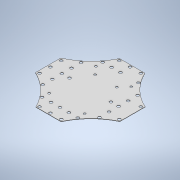
# Autodesk Inventor part: pixfalcon_acc_board_light
Saved by Autodesk Inventor 2020 (Build 240168000, 168)
## iProperties
Created: 2019-06-13
Part Number: pixfalcon_acc_board_light
Material: Generic
Document SubType Name: Modeling
Designer: amirt
Density: 1 g/cm^3
Appearance: Default
Author: amirt
Autodesk Inventor part; units mm, degrees
ref_plane "YZ Plane" through (0, 0, 0) normal (1, 0, 0) x (0, 1, 0)
ref_plane "XZ Plane" through (0, 0, 0) normal (0, 1, 0) x (-1, 0, 0)
ref_plane "XY Plane" through (0, 0, 0) normal (0, 0, 1) x (1, 0, 0)
sketch "Sketch1" plane through (25.3999, 76.2, 1203.3249) normal (0, 1, 0) x (-1, 0, 0)
  circle A0 centre (-1238.2523, -1095.3736) radius 57.1474 projected
  circle A1 centre (-1670.051, -1095.3758) radius 57.1513 projected
  circle A2 centre (-958.8491, -714.3774) radius 57.1526 projected
  circle A3 centre (-1314.4507, -714.3762) radius 57.1514 projected
  circle A4 centre (-1670.0504, -714.3731) radius 57.1481 projected
  circle A5 centre (-2101.8571, -1095.3735) radius 57.1571 projected
  circle A6 centre (-2381.2539, -714.3704) radius 57.1441 projected
  circle A7 centre (-2374.9001, -437.5189) radius 44.4462 projected
  circle A8 centre (-965.201, -437.5113) radius 44.4463 projected
  circle A9 centre (-1238.2504, -135.2557) radius 44.4509 projected
  circle A10 centre (-539.7501, -269.8758) radius 57.1508 projected
  circle A11 centre (-82.5498, 60.325) radius 57.1503 projected
  circle A12 centre (-82.5503, 492.1251) radius 57.1497 projected
  circle A13 centre (-82.5503, 923.9249) radius 57.1497 projected
  circle A14 centre (-539.7506, 1254.1242) radius 57.149 projected
  circle A15 centre (-539.7506, 873.1259) radius 57.149 projected
  circle A16 centre (-539.7488, 492.1268) radius 57.1522 projected
  circle A17 centre (-539.7501, 111.124) radius 57.151 projected
  circle A18 centre (-844.552, 492.1153) radius 57.1402 projected
  circle A19 centre (-965.2029, 1421.7493) radius 44.4342 projected
  circle A20 centre (-958.8546, 1698.6268) radius 57.1451 projected
  circle A21 centre (-1238.2501, 2079.6258) radius 57.1505 projected
  circle A22 centre (-1314.4494, 1698.6235) radius 57.1516 projected
  circle A23 centre (-1670.0494, 1698.6235) radius 57.1516 projected
  circle A24 centre (-2025.6555, 1698.6281) radius 57.1438 projected
  circle A25 centre (-2381.2575, 1698.6334) radius 57.1389 projected
  circle A26 centre (-2101.8503, 2079.6254) radius 57.1496 projected
  circle A27 centre (-1670.0543, 2079.6363) radius 57.1384 projected
  circle A28 centre (-2374.8997, 1421.7644) radius 44.4506 projected
  circle A29 centre (-2800.3552, 1254.1333) radius 57.1404 projected
  circle A30 centre (-3257.5497, 923.9267) radius 57.1482 projected
  circle A31 centre (-2800.3372, 873.132) radius 57.1356 projected
  circle A32 centre (-2495.5435, 492.1228) radius 57.157 projected
  circle A33 centre (-2800.3503, 492.134) radius 57.1411 projected
  circle A34 centre (-3257.5494, 60.3259) radius 57.1489 projected
  circle A35 centre (-2800.342, 111.1204) radius 57.1592 projected
  circle A36 centre (-2800.3554, -269.8798) radius 57.1572 projected
  circle A37 centre (-2101.8507, -135.2543) radius 44.4491 projected
  line L0 (-82.5503, 930.2676) -> (-82.5503, 923.9249)
  line L1 (22.2091, 981.2172) -> (-3340.1002, 981.2172)
  line L2 (-3340.1002, 981.2172) -> (-3340.1002, -24.9907)
  line L3 (-3340.1002, -24.9907) -> (22.2091, -24.9907)
  line L4 (22.2091, -24.9907) -> (22.2091, 981.2172)
  line L5 (-1168.7163, -1177.925) -> (-2174.6389, -1177.925)
  line L6 (-2174.6389, -1177.925) -> (-2174.6389, 2159.3417)
  line L7 (-2174.6389, 2159.3417) -> (-1168.7163, 2159.3417)
  line L8 (-1168.7163, 2159.3417) -> (-1168.7163, -1177.925)
  arc A38 (-1168.7163, 2159.3417) -> (22.2091, 981.2172) centre (1132.2663, 3294.3305) ccw
  arc A39 (-3340.1002, 981.2172) -> (-2174.6389, 2159.3417) centre (-4424.2857, 3219.2786) ccw
  arc A40 (-2174.6389, -1177.925) -> (-3340.1002, -24.9907) centre (-4329.0768, -2190.2423) ccw
  arc A41 (22.2091, -24.9907) -> (-1168.7163, -1177.925) centre (1000.6036, -2227.1762) ccw
  point P0 (25.3999, -1203.3249)
  point P1 (-1257.3, 1089.0251)
  point P2 (-1257.3, 263.5251)
  point P3 (-2082.8002, 1089.0251)
  point P4 (-2082.8002, 263.5251)
  point P5 (-2171.5581, -1177.8007)
  point P6 (-2174.6389, 981.2172)
  point P7 (-1168.7163, 981.2172)
  point P8 (-1168.7163, -24.9907)
  point P9 (-2174.6389, -24.9907)
  constraints: 18 end point, 8 point on circle, 4 centre point, 4 parallel, 2 horizontal, 2 perpendicular, 1 vertical
extrude "Extrusion2" add sketch "Sketch1" along normal blind 12.7
body "Solid2"
